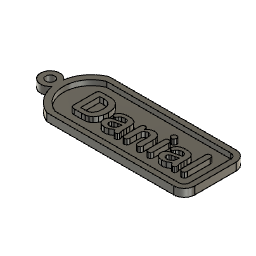
keytag (Autodesk Fusion 360 design; units mm, degrees)
Autodesk Fusion 360 part; units mm, degrees
sketch "Sketch1" plane through (0, 0, 0) normal (0, 0, 1) x (1, 0, 0)
  line L0 (0, 0) -> (48, 0)
  line L1 (50, 2) -> (50, 18)
  line L2 (48, 20) -> (0, 20)
  arc A0 (0, 20) -> (0, 0) centre (4.0751, 10) ccw
  arc A1 (50, 18) -> (48, 20) centre (48, 18) ccw
  arc A2 (48, 0) -> (50, 2) centre (48, 2) ccw
  line L3 (-1.2061, -2.0611) -> (48, -2.0611)
  arc A3 (48, -2.0611) -> (52.0611, 2) centre (48, 2) ccw
  line L4 (52.0611, 2) -> (52.0611, 18)
  arc A4 (52.0611, 18) -> (48, 22.0611) centre (48, 18) ccw
  line L5 (48, 22.0611) -> (-1.2061, 22.0611)
  circle A5 centre (-11.8904, 10) radius 1.75
  arc A6 (-8.8965, 12.2581) -> (-8.8965, 7.7419) centre (-11.8904, 10) ccw
  arc A7 (-1.2061, 22.0611) -> (-8.8965, 12.2581) centre (4.0751, 10) ccw
  arc A8 (-8.8965, 7.7419) -> (-1.2061, -2.0611) centre (4.0751, 10) ccw
  line L6 (2.8427, 15.3156) -> (5.6979, 15.3156)
  spline S0 degree 3 poles (5.6979, 15.3156) (6.0441, 15.3099) (6.6876, 15.2994) (7.3176, 15.1691) (7.6087, 15.109) knots 0 0 0 0 0.1036 0.192568 0.192568 0.192568 0.192568
  spline S1 degree 3 poles (7.6087, 15.109) (7.8694, 15.0239) (8.3973, 14.8517) (8.8338, 14.5082) (9.0547, 14.3343) knots 0 0 0 0 0.081585 0.165189 0.165189 0.165189 0.165189
  spline S2 degree 3 poles (9.0547, 14.3343) (9.5466, 13.7551) (10.6168, 12.4949) (10.6995, 10.8345) (10.7441, 9.9373) knots 0 0 0 0 0.22195 0.48287 0.48287 0.48287 0.48287
  spline S3 degree 3 poles (10.7441, 9.9373) (10.7383, 9.626) (10.7273, 9.0289) (10.6239, 8.4408) (10.5744, 8.1593) knots 0 0 0 0 0.093239 0.178848 0.178848 0.178848 0.178848
  spline S4 degree 3 poles (10.5744, 8.1593) (10.5119, 7.901) (10.3903, 7.3985) (10.1617, 6.9349) (10.0506, 6.7096) knots 0 0 0 0 0.079438 0.154562 0.154562 0.154562 0.154562
  spline S5 degree 3 poles (10.0506, 6.7096) (9.9238, 6.4997) (9.6688, 6.0775) (9.319, 5.7298) (9.1432, 5.555) knots 0 0 0 0 0.073279 0.147345 0.147345 0.147345 0.147345
  spline S6 degree 3 poles (9.1432, 5.555) (8.9954, 5.4314) (8.702, 5.1861) (8.3608, 5.0135) (8.1915, 4.9279) knots 0 0 0 0 0.057588 0.114305 0.114305 0.114305 0.114305
  spline S7 degree 3 poles (8.1915, 4.9279) (8.0147, 4.8548) (7.6559, 4.7065) (7.2746, 4.6331) (7.0812, 4.5959) knots 0 0 0 0 0.057227 0.116154 0.116154 0.116154 0.116154
  spline S8 degree 3 poles (7.0812, 4.5959) (6.8709, 4.568) (6.4265, 4.5089) (5.9783, 4.5031) (5.7421, 4.5) knots 0 0 0 0 0.063579 0.134352 0.134352 0.134352 0.134352
  line L7 (5.7421, 4.5) -> (2.887, 4.5)
  spline S9 degree 3 poles (2.887, 4.5) (2.7096, 4.5025) (2.3973, 4.5068) (2.1107, 4.6283) (1.9869, 4.6808) knots 0 0 0 0 0.052576 0.092569 0.092569 0.092569 0.092569
  spline S10 degree 3 poles (1.9869, 4.6808) (1.895, 4.7466) (1.7128, 4.8772) (1.6322, 5.0863) (1.5922, 5.1898) knots 0 0 0 0 0.03314 0.06568 0.06568 0.06568 0.06568
  spline S11 degree 3 poles (1.5922, 5.1898) (1.5654, 5.3151) (1.5053, 5.5958) (1.5019, 5.8829) (1.5, 6.0419) knots 0 0 0 0 0.038347 0.085896 0.085896 0.085896 0.085896
  line L8 (1.5, 6.0419) -> (1.5, 13.9728)
  spline S12 degree 3 poles (1.5, 13.9728) (1.5052, 14.1835) (1.5143, 14.5579) (1.7251, 14.8643) (1.8172, 14.9983) knots 0 0 0 0 0.061563 0.109398 0.109398 0.109398 0.109398
  spline S13 degree 3 poles (1.8172, 14.9983) (1.9512, 15.0905) (2.2577, 15.3012) (2.6321, 15.3104) (2.8427, 15.3156) knots 0 0 0 0 0.047836 0.109398 0.109398 0.109398 0.109398
  line L9 (3.6911, 13.5818) -> (3.6911, 6.2411)
  line L10 (3.6911, 6.2411) -> (5.3511, 6.2411)
  spline S14 degree 3 poles (5.3511, 6.2411) (5.5135, 6.2415) (5.7991, 6.2422) (6.084, 6.2621) (6.2069, 6.2706) knots 0 0 0 0 0.048698 0.085652 0.085652 0.085652 0.085652
  spline S15 degree 3 poles (6.2069, 6.2706) (6.3127, 6.2847) (6.5313, 6.3139) (6.7407, 6.3827) (6.8488, 6.4182) knots 0 0 0 0 0.031959 0.065985 0.065985 0.065985 0.065985
  spline S16 degree 3 poles (6.8488, 6.4182) (6.9548, 6.4607) (7.1625, 6.544) (7.3382, 6.6824) (7.4242, 6.7502) knots 0 0 0 0 0.034085 0.06674 0.06674 0.06674 0.06674
  spline S17 degree 3 poles (7.4242, 6.7502) (7.7435, 7.1552) (8.4763, 8.0849) (8.5065, 9.2785) (8.5235, 9.952) knots 0 0 0 0 0.151016 0.346618 0.346618 0.346618 0.346618
  spline S18 degree 3 poles (8.5235, 9.952) (8.5173, 10.4262) (8.5064, 11.2586) (8.1805, 12.0215) (8.0402, 12.3498) knots 0 0 0 0 0.14051 0.24667 0.24667 0.24667 0.24667
  spline S19 degree 3 poles (8.0402, 12.3498) (7.8781, 12.5884) (7.5732, 13.0375) (7.0799, 13.26) (6.8488, 13.3642) knots 0 0 0 0 0.084625 0.159221 0.159221 0.159221 0.159221
  spline S20 degree 3 poles (6.8488, 13.3642) (6.5893, 13.4276) (6.0273, 13.5648) (5.4486, 13.5759) (5.1372, 13.5818) knots 0 0 0 0 0.079888 0.173005 0.173005 0.173005 0.173005
  line L11 (5.1372, 13.5818) -> (3.6911, 13.5818)
  spline S21 degree 3 poles (17.6201, 5.4517) (17.3858, 5.2773) (16.9425, 4.9471) (16.4429, 4.711) (16.2072, 4.5996) knots 0 0 0 0 0.087359 0.165351 0.165351 0.165351 0.165351
  spline S22 degree 3 poles (16.2072, 4.5996) (15.9682, 4.5168) (15.4725, 4.3451) (14.9479, 4.3256) (14.6764, 4.3156) knots 0 0 0 0 0.075462 0.156466 0.156466 0.156466 0.156466
  spline S23 degree 3 poles (14.6764, 4.3156) (14.4304, 4.3261) (13.9578, 4.3463) (13.5235, 4.5325) (13.3152, 4.6217) knots 0 0 0 0 0.073163 0.140551 0.140551 0.140551 0.140551
  spline S24 degree 3 poles (13.3152, 4.6217) (13.1321, 4.731) (12.7731, 4.9452) (12.5304, 5.2852) (12.4115, 5.4517) knots 0 0 0 0 0.063213 0.123894 0.123894 0.123894 0.123894
  spline S25 degree 3 poles (12.4115, 5.4517) (12.3189, 5.63) (12.1339, 5.9866) (12.1075, 6.3874) (12.0942, 6.5879) knots 0 0 0 0 0.059554 0.119105 0.119105 0.119105 0.119105
  spline S26 degree 3 poles (12.0942, 6.5879) (12.1147, 6.8517) (12.1552, 7.3717) (12.4653, 7.7906) (12.618, 7.997) knots 0 0 0 0 0.077655 0.153066 0.153066 0.153066 0.153066
  spline S27 degree 3 poles (12.618, 7.997) (12.8156, 8.1766) (13.2306, 8.554) (13.7727, 8.7016) (14.0567, 8.779) knots 0 0 0 0 0.078958 0.165831 0.165831 0.165831 0.165831
  spline S28 degree 3 poles (14.0567, 8.779) (14.1679, 8.8032) (14.4847, 8.8719) (14.8023, 8.9364) (15.0084, 8.9782) knots 0 0 0 0 0.03415 0.097234 0.097234 0.097234 0.097234
  spline S29 degree 3 poles (15.0084, 8.9782) (15.2438, 9.0267) (15.6789, 9.1163) (16.1118, 9.2163) (16.3105, 9.2622) knots 0 0 0 0 0.072094 0.133281 0.133281 0.133281 0.133281
  spline S30 degree 3 poles (16.3105, 9.2622) (16.4993, 9.3088) (16.8934, 9.406) (17.2838, 9.5176) (17.4873, 9.5758) knots 0 0 0 0 0.05831 0.121788 0.121788 0.121788 0.121788
  spline S31 degree 3 poles (17.4873, 9.5758) (17.4729, 9.8115) (17.4477, 10.2255) (17.251, 10.5887) (17.1663, 10.7451) knots 0 0 0 0 0.069774 0.122545 0.122545 0.122545 0.122545
  spline S32 degree 3 poles (17.1663, 10.7451) (17.0262, 10.8529) (16.6843, 11.1161) (16.2475, 11.1171) (15.9896, 11.1177) knots 0 0 0 0 0.051802 0.126439 0.126439 0.126439 0.126439
  spline S33 degree 3 poles (15.9896, 11.1177) (15.7624, 11.115) (15.364, 11.1103) (14.994, 10.9659) (14.835, 10.9038) knots 0 0 0 0 0.067441 0.118271 0.118271 0.118271 0.118271
  spline S34 degree 3 poles (14.835, 10.9038) (14.7089, 10.8211) (14.4472, 10.6493) (14.2653, 10.3942) (14.171, 10.2619) knots 0 0 0 0 0.044819 0.093069 0.093069 0.093069 0.093069
  spline S35 degree 3 poles (14.171, 10.2619) (14.0941, 10.1423) (13.9703, 9.9496) (13.8323, 9.7668) (13.78, 9.6975) knots 0 0 0 0 0.042637 0.068681 0.068681 0.068681 0.068681
  spline S36 degree 3 poles (13.78, 9.6975) (13.7218, 9.6581) (13.5756, 9.5591) (13.3969, 9.5603) (13.2894, 9.561) knots 0 0 0 0 0.020692 0.051957 0.051957 0.051957 0.051957
  spline S37 degree 3 poles (13.2894, 9.561) (13.1805, 9.5698) (12.9644, 9.5872) (12.7896, 9.7152) (12.7029, 9.7787) knots 0 0 0 0 0.032096 0.063664 0.063664 0.063664 0.063664
  spline S38 degree 3 poles (12.7029, 9.7787) (12.6308, 9.8568) (12.4854, 10.0143) (12.4657, 10.2279) (12.4557, 10.3357) knots 0 0 0 0 0.030968 0.062473 0.062473 0.062473 0.062473
  spline S39 degree 3 poles (12.4557, 10.3357) (12.474, 10.5149) (12.5124, 10.8902) (12.7223, 11.2044) (12.832, 11.3685) knots 0 0 0 0 0.053219 0.111423 0.111423 0.111423 0.111423
  spline S40 degree 3 poles (12.832, 11.3685) (12.9845, 11.5321) (13.3169, 11.8887) (13.7633, 12.0873) (14.005, 12.1948) knots 0 0 0 0 0.066405 0.144792 0.144792 0.144792 0.144792
  spline S41 degree 3 poles (14.005, 12.1948) (14.3009, 12.2893) (14.9457, 12.4953) (15.6231, 12.511) (15.9896, 12.5195) knots 0 0 0 0 0.092707 0.202013 0.202013 0.202013 0.202013
  spline S42 degree 3 poles (15.9896, 12.5195) (16.3883, 12.514) (17.0996, 12.5043) (17.7789, 12.297) (18.0775, 12.2059) knots 0 0 0 0 0.118854 0.21206 0.21206 0.21206 0.21206
  spline S43 degree 3 poles (18.0775, 12.2059) (18.3107, 12.0893) (18.7652, 11.862) (19.0246, 11.4259) (19.1509, 11.2136) knots 0 0 0 0 0.076433 0.148947 0.148947 0.148947 0.148947
  spline S44 degree 3 poles (19.1509, 11.2136) (19.2421, 10.9529) (19.4455, 10.3712) (19.4577, 9.754) (19.4645, 9.4135) knots 0 0 0 0 0.082369 0.183745 0.183745 0.183745 0.183745
  spline S45 degree 3 poles (19.4645, 9.4135) (19.4644, 9.1952) (19.4642, 8.7944) (19.4618, 8.3935) (19.4608, 8.2109) knots 0 0 0 0 0.065476 0.120256 0.120256 0.120256 0.120256
  spline S46 degree 3 poles (19.4608, 8.2109) (19.4593, 8.0369) (19.4563, 7.6705) (19.452, 7.3041) (19.4497, 7.1117) knots 0 0 0 0 0.052199 0.109932 0.109932 0.109932 0.109932
  spline S47 degree 3 poles (19.4497, 7.1117) (19.4585, 6.9172) (19.4767, 6.5156) (19.583, 6.1277) (19.6378, 5.9276) knots 0 0 0 0 0.058197 0.120227 0.120227 0.120227 0.120227
  spline S48 degree 3 poles (19.6378, 5.9276) (19.6909, 5.7601) (19.7733, 5.5001) (19.8121, 5.2305) (19.826, 5.1345) knots 0 0 0 0 0.052558 0.081622 0.081622 0.081622 0.081622
  spline S49 degree 3 poles (19.826, 5.1345) (19.811, 5.0311) (19.7791, 4.8105) (19.6194, 4.6535) (19.5345, 4.5701) knots 0 0 0 0 0.030486 0.065096 0.065096 0.065096 0.065096
  spline S50 degree 3 poles (19.5345, 4.5701) (19.435, 4.4959) (19.2385, 4.3493) (18.9946, 4.3267) (18.8742, 4.3156) knots 0 0 0 0 0.036473 0.071999 0.071999 0.071999 0.071999
  spline S51 degree 3 poles (18.8742, 4.3156) (18.7677, 4.3313) (18.535, 4.3657) (18.3579, 4.5222) (18.2619, 4.607) knots 0 0 0 0 0.031651 0.069119 0.069119 0.069119 0.069119
  spline S52 degree 3 poles (18.2619, 4.607) (18.1546, 4.7233) (17.9138, 4.9842) (17.7248, 5.285) (17.6201, 5.4517) knots 0 0 0 0 0.047385 0.10629 0.10629 0.10629 0.10629
  spline S53 degree 3 poles (17.4873, 8.3659) (17.3069, 8.3077) (16.8838, 8.1711) (16.4492, 8.0769) (16.1999, 8.0228) knots 0 0 0 0 0.056824 0.133302 0.133302 0.133302 0.133302
  spline S54 degree 3 poles (16.1999, 8.0228) (15.9613, 7.9719) (15.5704, 7.8885) (15.1819, 7.794) (15.0305, 7.7572) knots 0 0 0 0 0.07317 0.119918 0.119918 0.119918 0.119918
  spline S55 degree 3 poles (15.0305, 7.7572) (14.9219, 7.7208) (14.6967, 7.6453) (14.5083, 7.5003) (14.4108, 7.4252) knots 0 0 0 0 0.034113 0.070742 0.070742 0.070742 0.070742
  spline S56 degree 3 poles (14.4108, 7.4252) (14.3248, 7.3319) (14.1455, 7.1375) (14.1259, 6.873) (14.1157, 6.7354) knots 0 0 0 0 0.036962 0.077025 0.077025 0.077025 0.077025
  spline S57 degree 3 poles (14.1157, 6.7354) (14.1307, 6.5881) (14.1609, 6.2909) (14.3613, 6.069) (14.4624, 5.9571) knots 0 0 0 0 0.043208 0.087218 0.087218 0.087218 0.087218
  spline S58 degree 3 poles (14.4624, 5.9571) (14.591, 5.8635) (14.8609, 5.6671) (15.195, 5.6468) (15.3699, 5.6362) knots 0 0 0 0 0.046704 0.098055 0.098055 0.098055 0.098055
  spline S59 degree 3 poles (15.3699, 5.6362) (15.5641, 5.6465) (15.9478, 5.6669) (16.2993, 5.8217) (16.4728, 5.8981) knots 0 0 0 0 0.057825 0.1142 0.1142 0.1142 0.1142
  spline S60 degree 3 poles (16.4728, 5.8981) (16.628, 5.9881) (16.9241, 6.16) (17.1207, 6.4398) (17.2143, 6.5731) knots 0 0 0 0 0.053077 0.101339 0.101339 0.101339 0.101339
  spline S61 degree 3 poles (17.2143, 6.5731) (17.2933, 6.7726) (17.4841, 7.2539) (17.4861, 7.7737) (17.4873, 8.0781) knots 0 0 0 0 0.063866 0.154132 0.154132 0.154132 0.154132
  line L12 (17.4873, 8.0781) -> (17.4873, 8.3659)
  line L13 (23.3377, 11.3907) -> (23.3377, 11.1472)
  spline S62 degree 3 poles (23.3377, 11.1472) (23.5125, 11.3619) (23.8439, 11.7688) (24.2892, 12.0456) (24.4997, 12.1764) knots 0 0 0 0 0.082375 0.15618 0.15618 0.15618 0.15618
  spline S63 degree 3 poles (24.4997, 12.1764) (24.7225, 12.2721) (25.185, 12.4709) (25.6884, 12.4931) (25.9494, 12.5047) knots 0 0 0 0 0.072115 0.149739 0.149739 0.149739 0.149739
  spline S64 degree 3 poles (25.9494, 12.5047) (26.2048, 12.4919) (26.7019, 12.4671) (27.1536, 12.2591) (27.3732, 12.1579) knots 0 0 0 0 0.075932 0.147757 0.147757 0.147757 0.147757
  spline S65 degree 3 poles (27.3732, 12.1579) (27.5688, 12.0308) (27.9585, 11.7775) (28.1933, 11.3765) (28.3102, 11.1767) knots 0 0 0 0 0.068947 0.13735 0.13735 0.13735 0.13735
  spline S66 degree 3 poles (28.3102, 11.1767) (28.3708, 11.0508) (28.493, 10.7969) (28.5432, 10.5196) (28.5684, 10.3799) knots 0 0 0 0 0.041728 0.0841 0.0841 0.0841 0.0841
  spline S67 degree 3 poles (28.5684, 10.3799) (28.5856, 10.2178) (28.624, 9.8549) (28.6262, 9.4899) (28.6274, 9.2881) knots 0 0 0 0 0.048893 0.109407 0.109407 0.109407 0.109407
  line L14 (28.6274, 9.2881) -> (28.6274, 5.5402)
  spline S68 degree 3 poles (28.6274, 5.5402) (28.6214, 5.3577) (28.6106, 5.0264) (28.4312, 4.7496) (28.3508, 4.6254) knots 0 0 0 0 0.053567 0.097183 0.097183 0.097183 0.097183
  spline S69 degree 3 poles (28.3508, 4.6254) (28.2503, 4.5351) (28.0458, 4.351) (27.7712, 4.3275) (27.6315, 4.3156) knots 0 0 0 0 0.039399 0.080256 0.080256 0.080256 0.080256
  spline S70 degree 3 poles (27.6315, 4.3156) (27.4894, 4.3278) (27.2101, 4.3519) (27.0029, 4.5403) (26.9011, 4.6328) knots 0 0 0 0 0.041526 0.081624 0.081624 0.081624 0.081624
  spline S71 degree 3 poles (26.9011, 4.6328) (26.8195, 4.7575) (26.64, 5.0318) (26.6275, 5.3608) (26.6207, 5.5402) knots 0 0 0 0 0.04391 0.096574 0.096574 0.096574 0.096574
  line L15 (26.6207, 5.5402) -> (26.6207, 8.897)
  spline S72 degree 3 poles (26.6207, 8.897) (26.6166, 9.1937) (26.6093, 9.7183) (26.4244, 10.2079) (26.3441, 10.4205) knots 0 0 0 0 0.088157 0.155876 0.155876 0.155876 0.155876
  spline S73 degree 3 poles (26.3441, 10.4205) (26.2172, 10.574) (25.9348, 10.9153) (25.4874, 10.9364) (25.2411, 10.948) knots 0 0 0 0 0.057269 0.127408 0.127408 0.127408 0.127408
  spline S74 degree 3 poles (25.2411, 10.948) (25.0653, 10.9344) (24.7122, 10.9071) (24.4111, 10.7207) (24.2599, 10.6271) knots 0 0 0 0 0.052081 0.104586 0.104586 0.104586 0.104586
  spline S75 degree 3 poles (24.2599, 10.6271) (24.1214, 10.508) (23.8377, 10.2641) (23.6875, 9.921) (23.6107, 9.7455) knots 0 0 0 0 0.054059 0.110742 0.110742 0.110742 0.110742
  spline S76 degree 3 poles (23.6107, 9.7455) (23.5681, 9.5309) (23.4583, 8.9764) (23.4613, 8.4104) (23.4631, 8.0634) knots 0 0 0 0 0.065496 0.169217 0.169217 0.169217 0.169217
  line L16 (23.4631, 8.0634) -> (23.4631, 5.5402)
  spline S77 degree 3 poles (23.4631, 5.5402) (23.4571, 5.3558) (23.4462, 5.0219) (23.2617, 4.7455) (23.1791, 4.6217) knots 0 0 0 0 0.054048 0.097849 0.097849 0.097849 0.097849
  spline S78 degree 3 poles (23.1791, 4.6217) (23.0759, 4.5324) (22.8652, 4.35) (22.587, 4.3272) (22.445, 4.3156) knots 0 0 0 0 0.039838 0.081402 0.081402 0.081402 0.081402
  spline S79 degree 3 poles (22.445, 4.3156) (22.3067, 4.3284) (22.0324, 4.3537) (21.8299, 4.5403) (21.7294, 4.6328) knots 0 0 0 0 0.04044 0.080242 0.080242 0.080242 0.080242
  spline S80 degree 3 poles (21.7294, 4.6328) (21.6478, 4.7575) (21.4683, 5.0318) (21.4558, 5.3608) (21.449, 5.5402) knots 0 0 0 0 0.04391 0.096574 0.096574 0.096574 0.096574
  line L17 (21.449, 5.5402) -> (21.449, 11.3612)
  spline S81 degree 3 poles (21.449, 11.3612) (21.4538, 11.5338) (21.4625, 11.8438) (21.6269, 12.1049) (21.6999, 12.2207) knots 0 0 0 0 0.05065 0.090994 0.090994 0.090994 0.090994
  spline S82 degree 3 poles (21.6999, 12.2207) (21.7938, 12.3035) (21.9895, 12.4759) (22.2504, 12.4949) (22.386, 12.5047) knots 0 0 0 0 0.036546 0.076105 0.076105 0.076105 0.076105
  spline S83 degree 3 poles (22.386, 12.5047) (22.4717, 12.4999) (22.6401, 12.4904) (22.7913, 12.4159) (22.8655, 12.3793) knots 0 0 0 0 0.025462 0.050021 0.050021 0.050021 0.050021
  spline S84 degree 3 poles (22.8655, 12.3793) (22.934, 12.3309) (23.0758, 12.2307) (23.1633, 12.0806) (23.2086, 12.003) knots 0 0 0 0 0.024845 0.051447 0.051447 0.051447 0.051447
  spline S85 degree 3 poles (23.2086, 12.003) (23.2462, 11.9114) (23.3266, 11.7154) (23.3338, 11.5035) (23.3377, 11.3907) knots 0 0 0 0 0.029486 0.063025 0.063025 0.063025 0.063025
  line L18 (32.6482, 11.3612) -> (32.6482, 5.5402)
  spline S86 degree 3 poles (32.6482, 5.5402) (32.6417, 5.3573) (32.6299, 5.0242) (32.4442, 4.7493) (32.3605, 4.6254) knots 0 0 0 0 0.053604 0.09762 0.09762 0.09762 0.09762
  spline S87 degree 3 poles (32.3605, 4.6254) (32.2572, 4.535) (32.0479, 4.3519) (31.7706, 4.3278) (31.6301, 4.3156) knots 0 0 0 0 0.040073 0.081201 0.081201 0.081201 0.081201
  spline S88 degree 3 poles (31.6301, 4.3156) (31.4902, 4.328) (31.2143, 4.3525) (31.011, 4.5403) (30.9108, 4.6328) knots 0 0 0 0 0.040892 0.080621 0.080621 0.080621 0.080621
  spline S89 degree 3 poles (30.9108, 4.6328) (30.8303, 4.7576) (30.6529, 5.0326) (30.6408, 5.3609) (30.6341, 5.5402) knots 0 0 0 0 0.043778 0.096431 0.096431 0.096431 0.096431
  line L19 (30.6341, 5.5402) -> (30.6341, 11.3021)
  spline S90 degree 3 poles (30.6341, 11.3021) (30.6401, 11.4824) (30.6509, 11.8092) (30.8303, 12.0805) (30.9108, 12.2022) knots 0 0 0 0 0.052836 0.095804 0.095804 0.095804 0.095804
  spline S91 degree 3 poles (30.9108, 12.2022) (31.0115, 12.2904) (31.2174, 12.4708) (31.4905, 12.4932) (31.6301, 12.5047) knots 0 0 0 0 0.039076 0.079898 0.079898 0.079898 0.079898
  spline S92 degree 3 poles (31.6301, 12.5047) (31.7704, 12.4929) (32.0464, 12.4698) (32.2569, 12.2904) (32.3605, 12.2022) knots 0 0 0 0 0.041094 0.080848 0.080848 0.080848 0.080848
  spline S93 degree 3 poles (32.3605, 12.2022) (32.4443, 12.086) (32.6246, 11.8358) (32.64, 11.5267) (32.6482, 11.3612) knots 0 0 0 0 0.042101 0.090592 0.090592 0.090592 0.090592
  spline S94 degree 3 poles (31.6522, 13.4417) (31.518, 13.4516) (31.2542, 13.4713) (31.0388, 13.6246) (30.9329, 13.6999) knots 0 0 0 0 0.03954 0.077736 0.077736 0.077736 0.077736
  spline S95 degree 3 poles (30.9329, 13.6999) (30.8458, 13.7985) (30.6623, 14.0065) (30.6438, 14.2843) (30.6341, 14.4302) knots 0 0 0 0 0.03839 0.080919 0.080919 0.080919 0.080919
  spline S96 degree 3 poles (30.6341, 14.4302) (30.6464, 14.5661) (30.6706, 14.835) (30.851, 15.0356) (30.9403, 15.1348) knots 0 0 0 0 0.039753 0.078691 0.078691 0.078691 0.078691
  spline S97 degree 3 poles (30.9403, 15.1348) (31.0462, 15.2155) (31.257, 15.3761) (31.5209, 15.3997) (31.6522, 15.4115) knots 0 0 0 0 0.039072 0.077782 0.077782 0.077782 0.077782
  spline S98 degree 3 poles (31.6522, 15.4115) (31.779, 15.401) (32.0327, 15.3799) (32.2413, 15.2338) (32.3457, 15.1606) knots 0 0 0 0 0.037417 0.074936 0.074936 0.074936 0.074936
  spline S99 degree 3 poles (32.3457, 15.1606) (32.4339, 15.0633) (32.6209, 14.8569) (32.6388, 14.5778) (32.6482, 14.4302) knots 0 0 0 0 0.038254 0.081163 0.081163 0.081163 0.081163
  spline S100 degree 3 poles (32.6482, 14.4302) (32.6384, 14.2861) (32.6196, 14.0105) (32.4391, 13.8026) (32.3531, 13.7036) knots 0 0 0 0 0.042059 0.080363 0.080363 0.080363 0.080363
  spline S101 degree 3 poles (32.3531, 13.7036) (32.2496, 13.6272) (32.041, 13.4732) (31.7825, 13.4522) (31.6522, 13.4417) knots 0 0 0 0 0.037784 0.076157 0.076157 0.076157 0.076157
  spline S102 degree 3 poles (39.8192, 5.4517) (39.585, 5.2773) (39.1417, 4.9471) (38.6421, 4.711) (38.4064, 4.5996) knots 0 0 0 0 0.087359 0.165351 0.165351 0.165351 0.165351
  spline S103 degree 3 poles (38.4064, 4.5996) (38.1674, 4.5168) (37.6717, 4.3451) (37.1471, 4.3256) (36.8756, 4.3156) knots 0 0 0 0 0.075462 0.156466 0.156466 0.156466 0.156466
  spline S104 degree 3 poles (36.8756, 4.3156) (36.6296, 4.3261) (36.157, 4.3463) (35.7227, 4.5325) (35.5144, 4.6217) knots 0 0 0 0 0.073163 0.140551 0.140551 0.140551 0.140551
  spline S105 degree 3 poles (35.5144, 4.6217) (35.3313, 4.731) (34.9723, 4.9452) (34.7296, 5.2852) (34.6107, 5.4517) knots 0 0 0 0 0.063213 0.123894 0.123894 0.123894 0.123894
  spline S106 degree 3 poles (34.6107, 5.4517) (34.5181, 5.63) (34.3331, 5.9866) (34.3066, 6.3874) (34.2934, 6.5879) knots 0 0 0 0 0.059554 0.119105 0.119105 0.119105 0.119105
  spline S107 degree 3 poles (34.2934, 6.5879) (34.3139, 6.8517) (34.3544, 7.3717) (34.6645, 7.7906) (34.8172, 7.997) knots 0 0 0 0 0.077655 0.153066 0.153066 0.153066 0.153066
  spline S108 degree 3 poles (34.8172, 7.997) (35.0148, 8.1766) (35.4298, 8.554) (35.9719, 8.7017) (36.2559, 8.779) knots 0 0 0 0 0.078957 0.16583 0.16583 0.16583 0.16583
  spline S109 degree 3 poles (36.2559, 8.779) (36.3671, 8.8032) (36.6838, 8.8719) (37.0015, 8.9364) (37.2076, 8.9782) knots 0 0 0 0 0.03415 0.097234 0.097234 0.097234 0.097234
  spline S110 degree 3 poles (37.2076, 8.9782) (37.443, 9.0267) (37.8781, 9.1163) (38.311, 9.2163) (38.5097, 9.2622) knots 0 0 0 0 0.072094 0.133281 0.133281 0.133281 0.133281
  spline S111 degree 3 poles (38.5097, 9.2622) (38.6985, 9.3088) (39.0926, 9.406) (39.483, 9.5176) (39.6865, 9.5758) knots 0 0 0 0 0.05831 0.121788 0.121788 0.121788 0.121788
  spline S112 degree 3 poles (39.6865, 9.5758) (39.6721, 9.8115) (39.6468, 10.2255) (39.4502, 10.5887) (39.3655, 10.7451) knots 0 0 0 0 0.069774 0.122545 0.122545 0.122545 0.122545
  spline S113 degree 3 poles (39.3655, 10.7451) (39.2254, 10.8529) (38.8835, 11.1161) (38.4467, 11.1171) (38.1888, 11.1177) knots 0 0 0 0 0.051803 0.126439 0.126439 0.126439 0.126439
  spline S114 degree 3 poles (38.1888, 11.1177) (37.9616, 11.115) (37.5632, 11.1103) (37.1932, 10.9659) (37.0342, 10.9038) knots 0 0 0 0 0.067441 0.118271 0.118271 0.118271 0.118271
  spline S115 degree 3 poles (37.0342, 10.9038) (36.9081, 10.8211) (36.6464, 10.6493) (36.4645, 10.3942) (36.3702, 10.2619) knots 0 0 0 0 0.044819 0.093069 0.093069 0.093069 0.093069
  spline S116 degree 3 poles (36.3702, 10.2619) (36.2933, 10.1423) (36.1695, 9.9496) (36.0315, 9.7668) (35.9792, 9.6975) knots 0 0 0 0 0.042637 0.068681 0.068681 0.068681 0.068681
  spline S117 degree 3 poles (35.9792, 9.6975) (35.921, 9.6581) (35.7748, 9.5591) (35.5961, 9.5603) (35.4886, 9.561) knots 0 0 0 0 0.020692 0.051957 0.051957 0.051957 0.051957
  spline S118 degree 3 poles (35.4886, 9.561) (35.3797, 9.5698) (35.1636, 9.5872) (34.9888, 9.7152) (34.9021, 9.7787) knots 0 0 0 0 0.032096 0.063664 0.063664 0.063664 0.063664
  spline S119 degree 3 poles (34.9021, 9.7787) (34.83, 9.8568) (34.6846, 10.0143) (34.6649, 10.2279) (34.6549, 10.3357) knots 0 0 0 0 0.030968 0.062473 0.062473 0.062473 0.062473
  spline S120 degree 3 poles (34.6549, 10.3357) (34.6732, 10.5149) (34.7116, 10.8902) (34.9215, 11.2044) (35.0312, 11.3685) knots 0 0 0 0 0.053219 0.111423 0.111423 0.111423 0.111423
  spline S121 degree 3 poles (35.0312, 11.3685) (35.1837, 11.5321) (35.5161, 11.8887) (35.9625, 12.0873) (36.2042, 12.1948) knots 0 0 0 0 0.066405 0.144792 0.144792 0.144792 0.144792
  spline S122 degree 3 poles (36.2042, 12.1948) (36.5001, 12.2893) (37.1449, 12.4953) (37.8223, 12.511) (38.1888, 12.5195) knots 0 0 0 0 0.092707 0.202013 0.202013 0.202013 0.202013
  spline S123 degree 3 poles (38.1888, 12.5195) (38.5875, 12.514) (39.2988, 12.5043) (39.9781, 12.297) (40.2767, 12.2059) knots 0 0 0 0 0.118854 0.21206 0.21206 0.21206 0.21206
  spline S124 degree 3 poles (40.2767, 12.2059) (40.5099, 12.0893) (40.9644, 11.862) (41.2238, 11.4259) (41.3501, 11.2136) knots 0 0 0 0 0.076433 0.148947 0.148947 0.148947 0.148947
  spline S125 degree 3 poles (41.3501, 11.2136) (41.4413, 10.9529) (41.6447, 10.3712) (41.6569, 9.754) (41.6636, 9.4135) knots 0 0 0 0 0.082369 0.183745 0.183745 0.183745 0.183745
  spline S126 degree 3 poles (41.6636, 9.4135) (41.6636, 9.1952) (41.6634, 8.7944) (41.661, 8.3935) (41.66, 8.2109) knots 0 0 0 0 0.065476 0.120256 0.120256 0.120256 0.120256
  spline S127 degree 3 poles (41.66, 8.2109) (41.6585, 8.0369) (41.6555, 7.6705) (41.6512, 7.3041) (41.6489, 7.1117) knots 0 0 0 0 0.052199 0.109932 0.109932 0.109932 0.109932
  spline S128 degree 3 poles (41.6489, 7.1117) (41.6577, 6.9172) (41.6758, 6.5156) (41.7822, 6.1277) (41.837, 5.9276) knots 0 0 0 0 0.058197 0.120227 0.120227 0.120227 0.120227
  spline S129 degree 3 poles (41.837, 5.9276) (41.8901, 5.7601) (41.9724, 5.5001) (42.0113, 5.2305) (42.0251, 5.1345) knots 0 0 0 0 0.052558 0.081622 0.081622 0.081622 0.081622
  spline S130 degree 3 poles (42.0251, 5.1345) (42.0102, 5.0311) (41.9783, 4.8105) (41.8186, 4.6535) (41.7337, 4.5701) knots 0 0 0 0 0.030486 0.065096 0.065096 0.065096 0.065096
  spline S131 degree 3 poles (41.7337, 4.5701) (41.6342, 4.4959) (41.4377, 4.3493) (41.1938, 4.3267) (41.0734, 4.3156) knots 0 0 0 0 0.036473 0.071999 0.071999 0.071999 0.071999
  spline S132 degree 3 poles (41.0734, 4.3156) (40.9669, 4.3313) (40.7342, 4.3657) (40.5571, 4.5222) (40.4611, 4.607) knots 0 0 0 0 0.031651 0.069119 0.069119 0.069119 0.069119
  spline S133 degree 3 poles (40.4611, 4.607) (40.3538, 4.7233) (40.113, 4.9842) (39.924, 5.285) (39.8192, 5.4517) knots 0 0 0 0 0.047385 0.10629 0.10629 0.10629 0.10629
  spline S134 degree 3 poles (39.6865, 8.3659) (39.5061, 8.3077) (39.083, 8.1711) (38.6484, 8.0769) (38.3991, 8.0228) knots 0 0 0 0 0.056824 0.133302 0.133302 0.133302 0.133302
  spline S135 degree 3 poles (38.3991, 8.0228) (38.1605, 7.9719) (37.7695, 7.8885) (37.3811, 7.794) (37.2297, 7.7572) knots 0 0 0 0 0.07317 0.119918 0.119918 0.119918 0.119918
  spline S136 degree 3 poles (37.2297, 7.7572) (37.1211, 7.7208) (36.8959, 7.6453) (36.7075, 7.5003) (36.61, 7.4252) knots 0 0 0 0 0.034113 0.070742 0.070742 0.070742 0.070742
  spline S137 degree 3 poles (36.61, 7.4252) (36.524, 7.3319) (36.3447, 7.1375) (36.3251, 6.873) (36.3149, 6.7354) knots 0 0 0 0 0.036962 0.077025 0.077025 0.077025 0.077025
  spline S138 degree 3 poles (36.3149, 6.7354) (36.3299, 6.5881) (36.3601, 6.2909) (36.5605, 6.069) (36.6616, 5.9571) knots 0 0 0 0 0.043208 0.087218 0.087218 0.087218 0.087218
  spline S139 degree 3 poles (36.6616, 5.9571) (36.7902, 5.8635) (37.0601, 5.6671) (37.3941, 5.6468) (37.5691, 5.6362) knots 0 0 0 0 0.046703 0.098055 0.098055 0.098055 0.098055
  spline S140 degree 3 poles (37.5691, 5.6362) (37.7633, 5.6465) (38.147, 5.6669) (38.4985, 5.8217) (38.672, 5.8981) knots 0 0 0 0 0.057825 0.1142 0.1142 0.1142 0.1142
  spline S141 degree 3 poles (38.672, 5.8981) (38.8272, 5.9881) (39.1233, 6.16) (39.3199, 6.4398) (39.4135, 6.5731) knots 0 0 0 0 0.053077 0.101339 0.101339 0.101339 0.101339
  spline S142 degree 3 poles (39.4135, 6.5731) (39.4925, 6.7726) (39.6833, 7.2539) (39.6853, 7.7737) (39.6865, 8.0781) knots 0 0 0 0 0.063866 0.154132 0.154132 0.154132 0.154132
  line L20 (39.6865, 8.0781) -> (39.6865, 8.3659)
  line L21 (43.7072, 5.5402) -> (43.7072, 14.2753)
  spline S143 degree 3 poles (43.7072, 14.2753) (43.7129, 14.4577) (43.7232, 14.7877) (43.8982, 15.0657) (43.9765, 15.1901) knots 0 0 0 0 0.053544 0.096898 0.096898 0.096898 0.096898
  spline S144 degree 3 poles (43.9765, 15.1901) (44.0764, 15.2805) (44.2824, 15.467) (44.5601, 15.4888) (44.7032, 15.5) knots 0 0 0 0 0.039251 0.081013 0.081013 0.081013 0.081013
  spline S145 degree 3 poles (44.7032, 15.5) (44.8469, 15.4887) (45.1267, 15.4667) (45.3381, 15.2831) (45.441, 15.1938) knots 0 0 0 0 0.042018 0.08178 0.08178 0.08178 0.08178
  spline S146 degree 3 poles (45.441, 15.1938) (45.5225, 15.07) (45.7049, 14.7929) (45.7155, 14.4597) (45.7213, 14.2753) knots 0 0 0 0 0.043667 0.097703 0.097703 0.097703 0.097703
  line L22 (45.7213, 14.2753) -> (45.7213, 5.5402)
  spline S147 degree 3 poles (45.7213, 5.5402) (45.7153, 5.3558) (45.7044, 5.0219) (45.5199, 4.7455) (45.4373, 4.6217) knots 0 0 0 0 0.054048 0.097849 0.097849 0.097849 0.097849
  spline S148 degree 3 poles (45.4373, 4.6217) (45.3342, 4.5324) (45.1234, 4.35) (44.8453, 4.3272) (44.7032, 4.3156) knots 0 0 0 0 0.039838 0.081402 0.081402 0.081402 0.081402
  spline S149 degree 3 poles (44.7032, 4.3156) (44.5633, 4.328) (44.2874, 4.3525) (44.0841, 4.5403) (43.9839, 4.6328) knots 0 0 0 0 0.040892 0.08062 0.08062 0.08062 0.08062
  spline S150 degree 3 poles (43.9839, 4.6328) (43.9034, 4.7576) (43.726, 5.0326) (43.7139, 5.3609) (43.7072, 5.5402) knots 0 0 0 0 0.043778 0.096431 0.096431 0.096431 0.096431
  dimension "d12" = 2
  constraint horizontal L0
  constraint vertical L1
  constraint horizontal L2
  constraint coincident L0.start A0.end
  constraint equal A1 A2
  constraint concentric A5 A6
  constraint coincident A6.end A7
  constraint parallel L0 L3
  constraint concentric A2 A3
  constraint parallel L1 L4
  constraint concentric A1 A4
  constraint parallel L2 L5
  constraint concentric A0 A7
  constraint tangent L3 A3
  constraint tangent A3 L4
  constraint tangent L4 A4
  constraint tangent A4 L5
  constraint concentric A7 A8
  measures "d12" radius of A1
extrude "Extrude1" add sketch "Sketch1" along normal blind 1 contours L0 L1 L2 A0 A1 A2 | L9 L10 S14 S15 S16 S17 S18 S19 S20 L11 | S53 S54 S55 S56 S57 S58 S59 S60 S61 L12 | S134 S135 S136 S137 S138 S139 S140 S141 S142 L20 makes body 1 at (6.3372, 9.925, 0) makes body 2 at (15.8329, 7.1968, 0) makes body 3 at (-1.2411, 10.0049, 0) makes body 4 at (38.0321, 7.1968, 0)
extrude "Extrude2" add sketch "Sketch1" along normal blind 3 bodies 1 2 3 4
